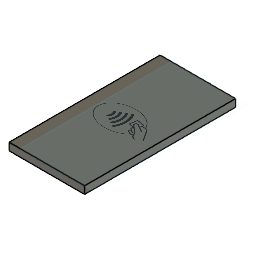
keychain (Autodesk Fusion 360 archive; units mm, degrees)
design "nfc"
part number: 2026-09-15-00-04-08-904
Autodesk Fusion 360 part; units mm, degrees
other "DerivedContext1"
sketch "sketch 234" plane through (0, 0, 15) normal (0, 0, 1) x (-1, 0, 0)
  arc A0 (-37.5, -25.5) -> (-40.5, -28.5) centre (-37.5, -28.5) ccw
  line L0 (-40.5, -28.5) -> (-40.5, -76.5)
  arc A1 (-40.5, -76.5) -> (-37.5, -79.5) centre (-37.5, -76.5) ccw
  line L1 (-37.5, -79.5) -> (-3.5, -79.5)
  arc A2 (-3.5, -79.5) -> (-0.5, -76.5) centre (-3.5, -76.5) ccw
  line L2 (-0.5, -76.5) -> (-0.5, -28.5)
  arc A3 (-0.5, -28.5) -> (-3.5, -25.5) centre (-3.5, -28.5) ccw
  line L3 (-3.5, -25.5) -> (-37.5, -25.5)
  line L4 (-15.5, -62.5) -> (-25.5, -62.5)
  line L5 (-25.5, -62.5) -> (-25.5, -42.5)
  line L6 (-25.5, -42.5) -> (-15.5, -42.5)
  line L7 (-15.5, -42.5) -> (-15.5, -62.5)
extrude "Extrude1" add sketch "sketch 234" along normal blind 1 contours L4 L5 L6 L7
sketch "Sketch1" plane through (0, 0, 16) normal (0, 0, 1) x (-1, 0, 0)
  line L0 (-15.5, -42.5) -> (-25.5, -42.5)
  line L1 (-25.5, -42.5) -> (-25.5, -62.5)
  line L2 (-25.5, -62.5) -> (-15.5, -62.5)
  line L3 (-15.5, -62.5) -> (-15.5, -42.5)
move_body "Move1" bodies 1 to x (1, 0, 0) y (0, 1, 0) z (0, 0, 1) at (-1.498, 0, 0)

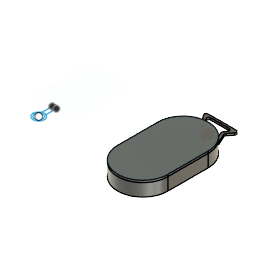
design "case"
part number: 2026-09-14-23-48-16-796
Autodesk Fusion 360 part; units mm, degrees
other "DerivedContext1"
sketch "Sketch1" plane through (0, 0, 0) normal (0, 0, 1) x (1, 0, 0)
  line L0 (2, 78) -> (39, 78)
  line L1 (39, 78) -> (39, 27)
  line L2 (39, 27) -> (2, 27)
  line L3 (2, 27) -> (2, 78)
  line L4 (3.5, 79.5) -> (37.5, 79.5)
  line L5 (40.5, 76.5) -> (40.5, 28.5)
  line L6 (37.5, 25.5) -> (3.5, 25.5)
  line L7 (0.5, 28.5) -> (0.5, 76.5)
  arc A0 (0.5, 28.5) -> (3.5, 25.5) centre (3.5, 28.5) ccw
  arc A1 (37.5, 25.5) -> (40.5, 28.5) centre (37.5, 28.5) ccw
  arc A2 (3.5, 79.5) -> (0.5, 76.5) centre (3.5, 76.5) ccw
  arc A3 (40.5, 76.5) -> (37.5, 79.5) centre (37.5, 76.5) ccw
  dimension "d4" = 3
  constraint horizontal L0
  constraint vertical L1
  constraint horizontal L2
  constraint vertical L3
  constraint horizontal L4
  constraint vertical L5
  constraint horizontal L6
  constraint vertical L7
  constraint tangent L6 A0
  constraint tangent L7 A0
  constraint tangent L5 A1
  constraint tangent L6 A1
  constraint equal A0 A1
  constraint tangent L4 A2
  constraint tangent L7 A2
  constraint equal A0 A2
  constraint tangent L4 A3
  constraint tangent L5 A3
  constraint equal A0 A3
  measures "d4" radius of A0
sketch "Sketch2" plane through (0, 0, 15) normal (0, 0, 1) x (-1, 0, 0)
  arc A0 (-37.5, -25.5) -> (-40.5, -28.5) centre (-37.5, -28.5) ccw
  line L0 (-40.5, -28.5) -> (-40.5, -76.5)
  arc A1 (-40.5, -76.5) -> (-37.5, -79.5) centre (-37.5, -76.5) ccw
  line L1 (-37.5, -79.5) -> (-3.5, -79.5)
  arc A2 (-3.5, -79.5) -> (-0.5, -76.5) centre (-3.5, -76.5) ccw
  line L2 (-0.5, -76.5) -> (-0.5, -28.5)
  arc A3 (-0.5, -28.5) -> (-3.5, -25.5) centre (-3.5, -28.5) ccw
  line L3 (-3.5, -25.5) -> (-37.5, -25.5)
  line L4 (-18.5, -25.5) -> (-22.5, -25.5)
  line L5 (-22.5, -25.5) -> (-22.5, -15.1235)
  line L6 (-18.5, -15.1235) -> (-18.5, -25.5)
  circle A4 centre (-20.5, -10) radius 5.5
  circle A5 centre (-20.5, -10) radius 4
  dimension "d19" = 11
  dimension "d20" = 8
  constraint coincident L3 L4.start
  constraint coincident L3 L4.end
  constraint perpendicular L3 L5
  constraint perpendicular L3 L6
  constraint concentric A4 A5
  constraint coincident L5.end A4
  constraint coincident L6.start A4
  measures "d19" diameter of A4
  measures "d20" diameter of A5
sketch "Sketch3" plane through (0, 0, 0) normal (0, 0, 1) x (1, 0, 0)
sketch "Sketch4" plane through (0, 0, 0) normal (0, 0, 1) x (1, 0, 0)
  line L0 (134, 25) -> (134, 65)
  line L1 (84, 65) -> (84, 25)
  arc A0 (109, 90) -> (84, 65) centre (109, 65) ccw
  arc A1 (134, 65) -> (109, 90) centre (109, 65) ccw
  arc A2 (84, 25) -> (109, 0) centre (109, 25) ccw
  arc A3 (109, 0) -> (134, 25) centre (109, 25) ccw
  line L2 (132, 25) -> (132, 65)
  line L3 (86, 65) -> (86, 25)
  arc A4 (132, 65) -> (109, 88) centre (109, 65) ccw
  arc A5 (109, 88) -> (86, 65) centre (109, 65) ccw
  arc A6 (86, 25) -> (109, 2) centre (109, 25) ccw
  arc A7 (109, 2) -> (132, 25) centre (109, 25) ccw
  point P0 (84, 0)
  point P1 (134, 0)
  point P2 (84, 90)
  dimension "d26" = 50
  dimension "d27" = 90
  dimension "d28" = 25
  dimension "d29" = 25
  dimension "d30" = 25
  dimension "d31" = 25
  dimension "d32" = 23
  dimension "d33" = 23
  dimension "d34" = 23
  dimension "d35" = 23
  constraint vertical L0
  constraint vertical L1
  constraint coincident P2 L1
  constraint tangent L1 A0
  constraint tangent L0 A1
  constraint coincident A0.start A1.end
  constraint coincident P0 L1
  constraint tangent L1 A2
  constraint coincident P1 L0
  constraint tangent L0 A3
  constraint coincident A2.end A3.start
  constraint vertical L2
  constraint vertical L3
  constraint tangent L2 A4
  constraint tangent L3 A5
  constraint coincident A4.end A5.start
  constraint tangent L3 A6
  constraint tangent L2 A7
  constraint coincident A6.end A7.start
  measures "d26" distance of P0 P1
  measures "d27" distance of P0 P2
  measures "d28" radius of A0
  measures "d29" radius of A1
  measures "d30" radius of A2
  measures "d31" radius of A3
  measures "d32" radius of A4
  measures "d33" radius of A5
  measures "d34" radius of A6
  measures "d35" radius of A7
extrude "Extrude8" add sketch "Sketch4" along normal blind 2 contours L0 L1 A0 A1 A2 A3 | L2 L3 A4 A5 A6 A7 makes body 1
extrude "Extrude9" add sketch "Sketch4" along normal blind 5 bodies 1
extrude "Extrude10" add sketch "Sketch4" along normal blind 12.5 bodies 1
extrude "Extrude11" add sketch "Sketch4" along normal blind 2 separate body contours L0 L1 A0 A1 A2 A3 | L2 L3 A4 A5 A6 A7 makes body 2
move_body "Move4" bodies 2 to x (1, 0, 0) y (0, 1, 0) z (0, 0, 1) at (0, 0, 12.5)
sketch "Sketch5" plane through (84, 0, 0) normal (-1, 0, 0) x (0, -1, 0)
  line L0 (-65, 0) -> (-25, 0)
  line L1 (-25, 0) -> (-25, 12.5)
  line L2 (-25, 12.5) -> (-65, 12.5)
  line L3 (-65, 12.5) -> (-65, 0)
  line L4 (-36.5, 6.5) -> (-28.5, 6.5)
  line L5 (-27.5, 5.5) -> (-27.5, 3.8)
  line L6 (-28.5, 2.8) -> (-36.5, 2.8)
  line L7 (-37.5, 3.8) -> (-37.5, 5.5)
  arc A0 (-27.5, 5.5) -> (-28.5, 6.5) centre (-28.5, 5.5) ccw
  arc A1 (-28.5, 2.8) -> (-27.5, 3.8) centre (-28.5, 3.8) ccw
  arc A2 (-37.5, 3.8) -> (-36.5, 2.8) centre (-36.5, 3.8) ccw
  arc A3 (-36.5, 6.5) -> (-37.5, 5.5) centre (-36.5, 5.5) ccw
  point P0 (-37.5, 6.5)
  point P1 (-27.5, 6.5)
  point P2 (-37.5, 2.8)
  dimension "d44" = 10
  dimension "d45" = 3.7
  dimension "d46" = 1
  constraint horizontal L4
  constraint vertical L5
  constraint horizontal L6
  constraint vertical L7
  constraint coincident P1 L4
  constraint coincident P1 L5
  constraint tangent L4 A0
  constraint tangent L5 A0
  constraint tangent L5 A1
  constraint tangent L6 A1
  constraint equal A0 A1
  constraint coincident P2 L6
  constraint coincident P2 L7
  constraint tangent L6 A2
  constraint tangent L7 A2
  constraint equal A0 A2
  constraint coincident P0 L4
  constraint coincident P0 L7
  constraint tangent L4 A3
  constraint tangent L7 A3
  constraint equal A0 A3
  measures "d44" distance of P0 P1
  measures "d45" distance of P0 P2
  measures "d46" radius of A0
extrude "Extrude12" cut sketch "Sketch5" against normal blind 2 contours L4 L5 L6 L7 A0 A1 A2 A3 bodies 1
sketch "Sketch6" plane through (0, 0, 14.5) normal (0, 0, 1) x (-1, 0, 0)
  arc A0 (-84, -25) -> (-134, -25) centre (-109, -25) ccw
  line L0 (-134, -25) -> (-134, -65)
  arc A1 (-134, -65) -> (-84, -65) centre (-109, -65) ccw
  line L1 (-84, -65) -> (-84, -25)
  line L2 (-125.0033, -84.2066) -> (-120.5129, -93.8936)
  line L3 (-120.7487, -95.9626) -> (-124.4894, -100.7721)
  line L4 (-122.9107, -104) -> (-109, -104)
  line L5 (-92.9967, -84.2066) -> (-97.4871, -93.8936)
  line L6 (-97.2513, -95.9626) -> (-93.5106, -100.7721)
  line L7 (-95.0893, -104) -> (-109, -104)
  line L8 (-96.9762, -86.9187) -> (-100.4296, -93.8545)
  line L9 (-100.1989, -95.9979) -> (-98.109, -98.6014)
  line L10 (-99.6686, -101.8534) -> (-118.0652, -101.8534)
  line L11 (-119.6809, -98.6746) -> (-117.7028, -95.9633)
  line L12 (-117.5133, -93.9237) -> (-120.7946, -87.0429)
  arc A2 (-100.4296, -93.8545) -> (-100.1989, -95.9979) centre (-98.6393, -94.7459) ccw
  arc A3 (-97.4871, -93.8936) -> (-97.2513, -95.9626) centre (-95.6726, -94.7347) ccw
  arc A4 (-117.7028, -95.9633) -> (-117.5133, -93.9237) centre (-119.3185, -94.7846) ccw
  arc A5 (-120.7487, -95.9626) -> (-120.5129, -93.8936) centre (-122.3274, -94.7347) ccw
  arc A6 (-124.4894, -100.7721) -> (-122.9107, -104) centre (-122.9107, -102) ccw
  arc A7 (-119.6809, -98.6746) -> (-118.0652, -101.8534) centre (-118.0652, -99.8534) ccw
  arc A8 (-99.6686, -101.8534) -> (-98.109, -98.6014) centre (-99.6686, -99.8534) ccw
  arc A9 (-95.0893, -104) -> (-93.5106, -100.7721) centre (-95.0893, -102) ccw
  dimension "d49" = 2
  constraint coincident A1 L2.start
  constraint horizontal L4
  constraint coincident A1 L8.start
  constraint horizontal L10
  constraint coincident A1 L12.end
  constraint tangent L8 A2
  constraint tangent L9 A2
  constraint tangent L5 A3
  constraint tangent L6 A3
  constraint equal A2 A3
  constraint tangent L11 A4
  constraint tangent L12 A4
  constraint equal A2 A4
  constraint tangent L2 A5
  constraint tangent L3 A5
  constraint equal A2 A5
  constraint tangent L3 A6
  constraint tangent L4 A6
  constraint equal A2 A6
  constraint tangent L10 A7
  constraint tangent L11 A7
  constraint equal A2 A7
  constraint tangent L9 A8
  constraint tangent L10 A8
  constraint equal A2 A8
  constraint tangent L6 A9
  constraint tangent L7 A9
  constraint equal A2 A9
  measures "d49" radius of A2
extrude "Extrude13" add sketch "Sketch6" against normal blind 2 separate body contours A1 L2 L3 L4 L5 L6 L7 L8 L9 L10 L11 L12 A2 A3 A4 A5 A6 A7 A8 A9 makes body 3
move_body "Move5" bodies 3 to x (1, 0, 0) y (0, 1, 0) z (0, 0, 1) at (0, 0, -8)
move_body "Move6" bodies 3 to x (1, 0, 0) y (0, 1, 0) z (0, 0, 1) at (0, 0, 1)
sketch "Sketch7" plane through (0, 0, 14.5) normal (0, 0, 1) x (-1, 0, 0)
  arc A0 (-84, -25) -> (-134, -25) centre (-109, -25) ccw
  line L0 (-134, -25) -> (-134, -65)
  arc A1 (-134, -65) -> (-84, -65) centre (-109, -65) ccw
  line L1 (-84, -65) -> (-84, -25)

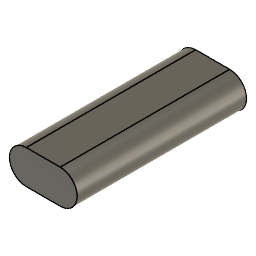
design "Untitled"
part number: 2026-09-14-23-44-04-987
Autodesk Fusion 360 part; units mm, degrees
sketch "Sketch1" plane through (0, 0, 0) normal (0, 0, 1) x (1, 0, 0)
  line L0 (0, 0) -> (20, 0)
  line L1 (20, 0) -> (20, 50)
  line L2 (20, 50) -> (0, 50)
  line L3 (0, 50) -> (0, 0)
  dimension "d1" = 20
  dimension "d2" = 50
  constraint horizontal L0
  constraint vertical L1
  constraint horizontal L2
  constraint vertical L3
  constraint coincident L0.start L3.end
  measures "d1" distance of L0.start L0.end
  measures "d2" distance of L0.start L2.end
extrude "Extrude1" add sketch "Sketch1" along normal blind 10
fillet "Fillet1" radius 5 4 edges at (20, 25, 10) (0, 25, 10) (20, 25, 0) (0, 25, 0)
move_body "Move1" bodies 1 to x (1, 0, 0) y (0, 1, 0) z (0, 0, 1) at (9, 0, 0)
move_body "Move2" bodies 1 to x (1, 0, 0) y (0, 1, 0) z (0, 0, 1) at (84, -7, 0)
move_body "Move3" bodies 1 to x (1, 0, 0) y (0, 1, 0) z (0, 0, 1) at (0, 0, 1)
